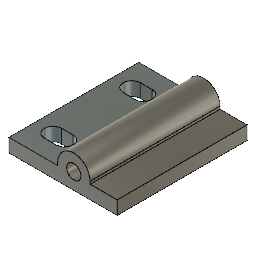
Rod Mount (Autodesk Fusion 360 design; units mm, degrees)
Autodesk Fusion 360 part; units mm, degrees
sketch "Sketch2" plane through (0, 0, 0) normal (0, 1, 0) x (1, 0, 0)
  line L0 (0, 0) -> (31.75, 0)
  line L1 (31.75, 0) -> (31.75, -9.525)
  line L2 (31.75, -9.525) -> (0, -9.525)
  line L3 (0, -9.525) -> (0, 0)
  circle A0 centre (19.05, -4.7625) radius 2.1
  line L4 (23.8125, 0) -> (14.2875, 0)
  line L5 (14.2875, 0) -> (14.2875, -9.525)
  line L6 (14.2875, -9.525) -> (23.8125, -9.525)
  line L7 (23.8125, -9.525) -> (23.8125, 0)
  line L8 (23.8125, 0) -> (14.2875, -9.525) construction
  line L9 (14.2875, 0) -> (23.8125, -9.525) construction
  line L10 (0, -4) -> (14.2875, -4)
  line L11 (23.8125, -4) -> (31.75, -4)
  point P0 (19.05, -4.7625)
  dimension "d1" = 31.75
  dimension "d2" = 9.525
  dimension "d3" = 4.2
  dimension "d4" = 4.7625
  dimension "d5" = 19.05
  dimension "d8" = 9.525
  dimension "d9" = 9.525
  dimension "d10" = 4
  dimension "d11" = 4
  constraint horizontal L0
  constraint vertical L1
  constraint horizontal L2
  constraint vertical L3
  constraint coincident L0.start L3.end
  constraint horizontal L4
  constraint perpendicular L4 L5
  constraint parallel L4 L6
  constraint parallel L5 L7
  constraint coincident L8 P0
  constraint coincident L9 P0
  constraint coincident P0 A0.centre
  constraint coincident L3 L10.start
  constraint coincident L5 L10.end
  constraint perpendicular L5 L10
  constraint coincident L7 L11.start
  constraint coincident L1 L11.end
  constraint perpendicular L1 L11
  measures "d1" distance of L0.start L0.end
  measures "d2" distance of L0.start L2.end
  measures "d3" diameter of A0
  measures "d4" distance of L0 P0
  measures "d5" distance of L3 P0
  measures "d8" distance of L5.end L6.end
  measures "d9" distance of L4.end L5.end
  measures "d10" distance of L0 L10
  measures "d11" distance of L0 L11
extrude "Extrude1" add sketch "Sketch2" along normal blind 38.1 contours L0 L3 L5 L10 | L0 L2 L4 L5 L6 L7 | L0 L1 L7 L11
fillet "Fillet1" radius 4.7625 2 edges at (14.2875, 19.05, 9.525) (23.8125, 19.05, 9.525)
sketch "Sketch3" plane through (0, 0, 4) normal (0, 0, 1) x (-1, 0, 0)
  line L0 (0, 0) -> (-14.2875, 0)
  line L1 (-14.2875, 0) -> (-14.2875, -38.1)
  line L2 (-14.2875, -38.1) -> (0, -38.1)
  line L3 (0, -38.1) -> (0, 0)
sketch "Sketch4" plane through (0, 0, 4) normal (0, 0, 1) x (-1, 0, 0)
sketch "Sketch5" plane through (0, 0, 4) normal (0, 0, 1) x (-1, 0, 0)
  line L0 (-14.2875, -38.1) -> (0, -38.1) construction
  line L1 (0, -38.1) -> (0, 0) construction
  line L2 (0, 0) -> (-14.2875, 0) construction
  line L3 (-14.2875, 0) -> (-14.2875, -38.1) construction
  line L4 (-7.1437, -38.1) -> (-7.1437, 0) construction
  line L5 (-7.1437, -27.2901) -> (0, -27.2901) construction
  line L6 (-7.1437, -27.2901) -> (-14.2875, -27.2901) construction
  line L7 (-5.4299, -28.1) -> (-8.8576, -28.1)
  arc A0 (-8.8576, -28.1) -> (-8.8576, -33.1) centre (-8.8576, -30.6) ccw
  line L8 (-8.8576, -33.1) -> (-5.4299, -33.1)
  arc A1 (-5.4299, -33.1) -> (-5.4299, -28.1) centre (-5.4299, -30.6) ccw
  line L9 (-5.4299, -30.6) -> (-8.8576, -30.6) construction
  line L10 (-5.4437, -5) -> (-8.8438, -5)
  arc A2 (-8.8438, -5) -> (-8.8438, -10) centre (-8.8438, -7.5) ccw
  line L11 (-8.8438, -10) -> (-5.4437, -10)
  arc A3 (-5.4437, -10) -> (-5.4437, -5) centre (-5.4437, -7.5) ccw
  line L12 (-5.4437, -7.5) -> (-8.8438, -7.5) construction
  point P0 (0, -38.1)
  point P1 (-14.2875, -38.1)
  point P2 (-14.2875, 0)
  point P3 (-7.1437, -30.6)
  point P4 (-7.1438, -7.5)
  dimension "d14" = 5
  dimension "d16" = 5
  dimension "d19" = 7.5
  dimension "d20" = 7.5
  constraint horizontal L0
  constraint vertical L1
  constraint horizontal L2
  constraint vertical L3
  constraint coincident L1.end L2.start
  constraint coincident P1 L0.start
  constraint coincident L0 L4.start
  constraint coincident L2 L4.end
  constraint perpendicular L2 L4
  constraint coincident L4 L5.start
  constraint coincident L1 L5.end
  constraint perpendicular L1 L5
  constraint coincident L3 L6.end
  constraint perpendicular L3 L6
  constraint equal L5 L6
  constraint tangent L7 A0
  constraint tangent A0 L8
  constraint parallel L7 L8
  constraint tangent L8 A1
  constraint tangent L7 A1
  constraint perpendicular L4 L9
  constraint coincident L4 P3
  constraint midpoint L9 P3
  constraint tangent L10 A2
  constraint tangent A2 L11
  constraint parallel L10 L11
  constraint tangent L11 A3
  constraint tangent L10 A3
  constraint perpendicular L4 L12
  constraint coincident L4 P4
  constraint midpoint L12 P4
  measures "d14" diameter of A0
  measures "d16" diameter of A2
  measures "d19" distance of L2 P4
  measures "d20" distance of L0 P3
extrude "Extrude2" cut sketch "Sketch5" against normal blind 4
named bodies: "Rod mount"
